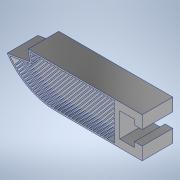
# Autodesk Inventor part: Finray_9_Kerbe_10deg
Saved by Autodesk Inventor 2022 (Build 260153000, 153)
## iProperties
Created: 2022-02-28
Part Number: Finray_9_Kerbe_10deg
Material: Generic
Document SubType Name: Modeling
Designer: richa
Density: 1 g/cm^3
Appearance: Aluminum - Flat
Author: richa
Autodesk Inventor part; units mm, degrees
ref_plane "YZ Plane" through (0, 0, 0) normal (1, 0, 0) x (0, 1, 0)
ref_plane "XZ Plane" through (0, 0, 0) normal (0, 1, 0) x (-1, 0, 0)
ref_plane "XY Plane" through (0, 0, 0) normal (0, 0, 1) x (1, 0, 0)
sketch "Sketch5" plane through (0, 0, 0) normal (0, 0, 1) x (1, 0, 0)
  line L0 (52.8, -15.6) -> (52.8, -10.6)
  line L1 (52.8, -10.6) -> (49.8, -10.6)
  line L2 (49.8, -10.6) -> (49.8, -12.6)
  line L3 (44, -12.6) -> (44, -3)
  line L4 (49.8, -3) -> (49.8, -5)
  line L5 (49.8, -5) -> (52.8, -5)
  line L6 (52.8, -5) -> (52.8, 0)
  line L7 (52.8, 0) -> (7.8, 0)
  line L8 (44, -3) -> (49.8, -3)
  line L9 (44, -12.6) -> (49.8, -12.6)
  line L10 (52.8, -15.6) -> (7.8, -15.6)
  line L11 (7.8, -15.6) -> (0, -15.6)
  line L12 (0, -15.6) -> (0, 0)
  line L13 (0, 0) -> (7.8, 0)
  point P0 (7.8, 0)
  dimension "d41" = 5.8
  dimension "d48" = 44
  dimension "d50" = 3
  dimension "d63" = 45
  dimension "d71" = 0
  dimension "d87" = 5.6
  dimension "d88" = 9.6
  dimension "d97" = 15.6
  constraints: 28 end point, 8 perpendicular, 4 collinear, 3 parallel, 2 horizontal, 1 vertical
  measures "d41" distance between parallel lines of L2 L3
  measures "d48" distance from line of L3 L12.end
  measures "d50" distance of L4.end L5.end
  measures "d63" distance of L0.start L10.end
  measures "d71" distance from line of L12.end L7
  measures "d87" distance from line of L0.end L5
  measures "d88" distance of L3.start L3.end
  measures "d97" distance of L11.end L12.end
extrude "Extrusion2" add sketch "Sketch5" along normal blind 12
sketch "Sketch8" plane through (0, 0, 0) normal (0, 0, -1) x (-1, 0, 0)
  line L0 (-8.1687, 0) -> (-8.8633, -3.9392)
  line L1 (-7.8, 0) -> (-1.143, 0) construction
  line L2 (0, -5.5021) -> (-8.8633, -3.9392)
  line L3 (-7.8, 0) -> (-8.1687, 0)
  line L4 (0, 0) -> (0, -15.6) projected
  line L5 (-52.8, 0) -> (0, 0) projected
  line L6 (-7.8, 0) -> (0, 0)
  line L7 (0, 0) -> (0, -5.5021)
  dimension "d80" = 100
  dimension "d95" = 4
  dimension "d96" = 9
  constraints: 12 end point, 2 collinear, 2 perpendicular, 1 horizontal, 1 point on line
  measures "d80" angle of L0 L1
  measures "d95" distance of L0.start L0.end
  measures "d96" distance of L2.start L0.end
extrude "Extrusion5" cut sketch "Sketch8" against normal through all
fillet "Fillet2" radius 23 1 edges at (0, -15.6, 6)
shell "Shell1" thickness 0.62 removed faces 1 at (23.9679, -7.5131, 12)
sketch "Sketch13" plane through (0, 0, 12) normal (0, 0, 1) x (1, 0, 0)
  line L0 (19.0404, -15.6) -> (52.8, -15.6) projected
  line L1 (42.0526, -15.6) -> (42.0526, 0)
  line L2 (52.8, 0) -> (8.1687, 0) projected
  line L3 (52.8, 0) -> (8.1687, 0) projected
  line L4 (52.8, -5) -> (52.8, 0) projected
  line L5 (49.8, -5) -> (52.8, -5) projected
  line L6 (49.8, -3) -> (49.8, -5) projected
  line L7 (44, -3) -> (49.8, -3) projected
  line L8 (44, -12.6) -> (44, -3) projected
  line L9 (49.8, -12.6) -> (44, -12.6) projected
  line L10 (49.8, -10.6) -> (49.8, -12.6) projected
  line L11 (52.8, -10.6) -> (49.8, -10.6) projected
  line L12 (52.8, -15.6) -> (52.8, -10.6) projected
  line L13 (42.0526, 0) -> (52.8, 0)
  line L14 (52.8, -5) -> (52.8, 0) projected
  line L15 (52.8, -5) -> (52.8, 0)
  line L16 (52.8, 0) -> (52.8, -5)
  line L17 (44, -12.6) -> (44, -3) projected
  line L18 (44, -3) -> (44, -12.6)
  line L19 (49.8, -12.6) -> (44, -12.6) projected
  line L20 (44, -12.6) -> (49.8, -12.6)
  line L21 (43.38, -13.22) -> (50.42, -13.22) projected
  line L22 (52.8, -10.6) -> (52.8, -15.6)
  line L23 (52.8, -15.6) -> (42.0526, -15.6)
  line L24 (44, -3) -> (49.8, -3) projected
  line L25 (44, -3) -> (49.8, -3)
  line L26 (49.8, -3) -> (49.8, -5)
  line L27 (49.8, -5) -> (52.8, -5)
  line L28 (52.8, -10.6) -> (49.8, -10.6)
  line L29 (49.8, -10.6) -> (49.8, -12.6)
  point P0 (0, 0)
  dimension "d102" = 10.7474
  constraints: 26 end point, 10 collinear, 2 point on line, 2 vertical, 1 parallel
  measures "d102" distance between parallel lines of L4 L1
extrude "Extrusion7" add sketch "Sketch13" against normal blind 12
sketch "Sketch14" plane through (8.9076, -0.62, 0.62) normal (0, 0, 1) x (1, 0, 0)
  line L0 (33.145, -14.36) -> (33.145, 0) projected
  line L1 (33.145, 0) -> (0, 0) projected
  line L2 (0.6739, -3.8221) -> (0, 0) projected
  line L3 (-7.835, -5.3225) -> (0.6739, -3.8221) projected
  arc A0 (-7.835, -5.3225) -> (10.1328, -14.36) centre (10.1328, 8.02) ccw projected
  line L4 (10.1328, -14.36) -> (33.145, -14.36) projected
  point P0 (-8.9076, 0.62)
extrude "Extrusion8" cut sketch "Sketch14" against normal blind 12
sketch "Sketch15" plane through (0, 0, 12) normal (0, 0, 1) x (1, 0, 0)
  line L0 (42.0526, -0.62) -> (8.9076, -0.62) construction
  line L1 (19.0404, -14.98) -> (42.0526, -14.98) projected
  line L2 (48.3066, -0.62) -> (36.2572, -14.98)
  line L3 (35.7611, -14.98) -> (47.8106, -0.62)
  line L4 (44.1485, -0.62) -> (32.099, -14.98)
  line L5 (31.6029, -14.98) -> (43.6524, -0.62)
  line L6 (39.9903, -0.62) -> (27.9408, -14.98)
  line L7 (27.4448, -14.98) -> (39.4943, -0.62)
  line L8 (35.8321, -0.62) -> (23.7827, -14.98)
  line L9 (23.2866, -14.98) -> (35.3361, -0.62)
  line L10 (31.674, -0.62) -> (19.6245, -14.98)
  line L11 (19.1285, -14.98) -> (31.1779, -0.62)
  line L12 (27.5158, -0.62) -> (15.6793, -14.7262)
  line L13 (15.2426, -14.6554) -> (27.0198, -0.62)
  line L14 (23.3577, -0.62) -> (11.7759, -14.4226)
  line L15 (19.1995, -0.62) -> (8.6931, -13.141)
  line L16 (8.3466, -12.9628) -> (18.7034, -0.62)
  arc A0 (1.0726, -5.9425) -> (19.0404, -14.98) centre (19.0404, 7.4) ccw projected
  line L17 (42.0526, -0.62) -> (42.0526, -14.98) projected
  line L18 (1.0726, -5.9425) -> (9.5815, -4.4421) projected
  arc A1 (0, -5.5021) -> (19.0404, -15.6) centre (19.0404, 7.4) ccw projected
  line L19 (10.3871, -0.62) -> (3.5571, -8.7596)
  line L20 (3.8342, -9.0206) -> (10.8832, -0.62)
  line L21 (14.5453, -0.62) -> (6.0082, -10.7941)
  line L22 (6.3201, -11.0135) -> (15.0413, -0.62)
  line L23 (42.0526, -14.98) -> (19.0404, -14.98) projected
  line L24 (38.5332, -14.98) -> (38.8243, -15.2243)
  line L25 (38.8243, -15.2243) -> (51.0787, -0.62)
  line L26 (51.0787, -0.62) -> (50.5827, -0.62)
  line L27 (50.5827, -0.62) -> (38.5332, -14.98)
  line L28 (8.9076, -0.62) -> (42.0526, -0.62) projected
  line L29 (46.4245, -0.62) -> (46.9206, -0.62)
  line L30 (46.9206, -0.62) -> (34.8711, -14.98)
  line L31 (34.8711, -14.98) -> (34.3751, -14.98)
  line L32 (34.3751, -14.98) -> (46.4245, -0.62)
  line L33 (42.2664, -0.62) -> (42.7624, -0.62)
  line L34 (42.7624, -0.62) -> (30.7129, -14.98)
  line L35 (30.7129, -14.98) -> (30.2169, -14.98)
  line L36 (30.2169, -14.98) -> (42.2664, -0.62)
  line L37 (38.1082, -0.62) -> (38.6043, -0.62)
  line L38 (38.6043, -0.62) -> (26.5548, -14.98)
  line L39 (26.5548, -14.98) -> (26.0587, -14.98)
  line L40 (26.0587, -14.98) -> (38.1082, -0.62)
  line L41 (33.95, -0.62) -> (34.4461, -0.62)
  line L42 (34.4461, -0.62) -> (22.3966, -14.98)
  line L43 (22.3966, -14.98) -> (21.9006, -14.98)
  line L44 (21.9006, -14.98) -> (33.95, -0.62)
  line L45 (29.7919, -0.62) -> (30.2879, -0.62)
  line L46 (30.2879, -0.62) -> (18.2385, -14.98)
  line L47 (18.2385, -14.98) -> (17.7424, -14.98)
  line L48 (17.7424, -14.98) -> (29.7919, -0.62)
  line L49 (25.6337, -0.62) -> (26.1298, -0.62)
  line L50 (26.1298, -0.62) -> (14.4751, -14.5094)
  line L51 (14.4751, -14.5094) -> (13.9791, -14.5094)
  line L52 (13.9791, -14.5094) -> (25.6337, -0.62)
  line L53 (21.4755, -0.62) -> (21.9716, -0.62)
  line L54 (21.9716, -0.62) -> (11.1333, -13.5366)
  line L55 (11.1333, -13.5366) -> (10.6372, -13.5366)
  line L56 (10.6372, -13.5366) -> (21.4755, -0.62)
  line L57 (17.3174, -0.62) -> (17.8134, -0.62)
  line L58 (17.8134, -0.62) -> (8.1413, -12.1467)
  line L59 (8.1413, -12.1467) -> (7.6453, -12.1467)
  line L60 (7.6453, -12.1467) -> (17.3174, -0.62)
  line L61 (9.4971, -0.62) -> (3.0705, -8.2789)
  line L62 (2.8052, -8.004) -> (9.001, -0.62)
  line L63 (10.5986, -4.2628) -> (10.1025, -4.2628)
  line L64 (13.1592, -0.62) -> (5.1587, -10.1546)
  line L65 (5.459, -10.3879) -> (13.6553, -0.62)
  line L66 (49.1966, -0.62) -> (49.6927, -0.62)
  line L67 (49.6927, -0.62) -> (37.6432, -14.98)
  line L68 (37.6432, -14.98) -> (37.1472, -14.98)
  line L69 (37.1472, -14.98) -> (49.1966, -0.62)
  line L70 (45.0385, -0.62) -> (45.5345, -0.62)
  line L71 (45.5345, -0.62) -> (33.4851, -14.98)
  line L72 (33.4851, -14.98) -> (32.989, -14.98)
  line L73 (32.989, -14.98) -> (45.0385, -0.62)
  line L74 (40.8803, -0.62) -> (41.3764, -0.62)
  line L75 (41.3764, -0.62) -> (29.3269, -14.98)
  line L76 (29.3269, -14.98) -> (28.8308, -14.98)
  line L77 (28.8308, -14.98) -> (40.8803, -0.62)
  line L78 (36.7221, -0.62) -> (37.2182, -0.62)
  line L79 (37.2182, -0.62) -> (25.1687, -14.98)
  line L80 (25.1687, -14.98) -> (24.6727, -14.98)
  line L81 (24.6727, -14.98) -> (36.7221, -0.62)
  line L82 (32.564, -0.62) -> (33.06, -0.62)
  line L83 (33.06, -0.62) -> (21.0106, -14.98)
  line L84 (21.0106, -14.98) -> (20.5145, -14.98)
  line L85 (20.5145, -14.98) -> (32.564, -0.62)
  line L86 (28.4058, -0.62) -> (28.9019, -0.62)
  line L87 (28.9019, -0.62) -> (16.8524, -14.98)
  line L88 (16.8524, -14.98) -> (16.3563, -14.98)
  line L89 (16.3563, -14.98) -> (28.4058, -0.62)
  line L90 (24.2477, -0.62) -> (24.7437, -0.62)
  line L91 (24.7437, -0.62) -> (13.3184, -14.2362)
  line L92 (13.3184, -14.2362) -> (12.8223, -14.2362)
  line L93 (12.8223, -14.2362) -> (24.2477, -0.62)
  line L94 (20.0895, -0.62) -> (20.5855, -0.62)
  line L95 (20.5855, -0.62) -> (10.0997, -13.1165)
  line L96 (10.0997, -13.1165) -> (9.6036, -13.1165)
  line L97 (9.6036, -13.1165) -> (20.0895, -0.62)
  line L98 (8.9718, -4.5497) -> (8.4758, -4.5497)
  line L99 (11.7732, -0.62) -> (4.3417, -9.4764)
  line L100 (4.6304, -9.7236) -> (12.2692, -0.62)
  line L101 (16.4274, -0.62) -> (15.9313, -0.62)
  line L102 (15.9313, -0.62) -> (6.8903, -11.3947)
  line L103 (7.214, -11.6) -> (16.4274, -0.62)
  line L104 (8.9076, -0.62) -> (-0.0004, -0.62) construction
  line L105 (47.8106, -0.62) -> (48.3066, -0.62)
  line L106 (11.8171, -13.7823) -> (22.8616, -0.62)
  point P0 (0, 0)
  point P1 (33.931, -17.161)
  point P2 (38.8393, -6.356)
  point P3 (29.043, -18.6221)
  point P4 (39.2193, -6.4943)
  point P5 (28.6321, -18.5205)
  point P6 (34.7397, -6.2863)
  point P7 (25.0778, -18.392)
  point P8 (24.4739, -18.5205)
  point P9 (27.5179, -9.9373)
  point P10 (28.1855, -9.733)
  point P11 (24.5233, -8.5506)
  point P12 (24.9033, -8.6889)
  point P13 (21.5288, -7.1639)
  point P14 (21.9088, -7.3022)
  point P15 (18.1464, -6.2394)
  point P16 (18.5264, -6.3777)
  point P17 (13.7227, -6.5558)
  point P18 (14.1901, -6.59)
  point P19 (7.3451, -4.8365)
  point P20 (4.128, -8.0793)
  point P21 (4.3811, -12.7332)
  point P22 (4.8055, -12.8186)
  point P23 (35.7611, -14.98)
  point P24 (31.6029, -14.98)
  point P25 (32.099, -14.98)
  point P26 (29.4219, -14.98)
  point P27 (27.9408, -14.98)
  point P28 (25.0643, -14.98)
  point P29 (23.7827, -14.98)
  point P30 (20.6649, -14.98)
  point P31 (21.1037, -14.98)
  point P32 (19.6462, -14.98)
  point P33 (20.0321, -14.98)
  point P34 (8.7548, -12.4764)
  point P35 (9.1029, -12.6527)
  point P36 (5.1362, -5.226)
  point P37 (3.0438, -8.3108)
  point P38 (1.8569, -9.134)
  point P39 (6.3464, -8.7392)
  point P40 (6.7558, -8.8424)
  point P41 (38.5332, -14.98)
  point P42 (39.0293, -14.98)
  point P43 (34.3751, -14.98)
  point P44 (34.8711, -14.98)
  point P45 (41.7215, -0.62)
  point P46 (41.1434, -0.62)
  point P47 (30.7129, -14.98)
  point P48 (41.6394, -0.62)
  point P49 (38.1082, -0.62)
  point P50 (26.5548, -14.98)
  point P51 (38.6043, -0.62)
  point P52 (33.95, -0.62)
  point P53 (22.3966, -14.98)
  point P54 (34.4461, -0.62)
  point P55 (29.7919, -0.62)
  point P56 (19.1984, -14.98)
  point P57 (19.0819, -14.98)
  point P58 (30.2879, -0.62)
  point P59 (26.1298, -0.62)
  point P60 (21.9716, -0.62)
  point P61 (17.8134, -0.62)
  point P62 (3.8395, -10.0749)
  point P63 (4.3026, -10.1142)
  point P64 (4.8631, -13.8106)
  point P65 (5.3932, -13.77)
  point P66 (37.6432, -14.98)
  point P67 (40.9208, -0.62)
  point P68 (32.989, -14.98)
  point P69 (33.4851, -14.98)
  point P70 (40.3355, -0.62)
  point P71 (29.3269, -14.98)
  point P72 (41.3764, -0.62)
  point P73 (25.1687, -14.98)
  point P74 (37.2182, -0.62)
  point P75 (21.0106, -14.98)
  point P76 (33.06, -0.62)
  point P77 (19.6871, -14.98)
  point P78 (19.1528, -14.98)
  point P79 (28.9019, -0.62)
  point P80 (24.7437, -0.62)
  point P81 (20.5855, -0.62)
  point P82 (15.9313, -0.62)
  point P83 (5.7184, -5.1233)
  point P84 (6.7629, -4.9391)
  point P85 (8.3897, -4.6523)
  point P86 (8.6984, -4.5979)
  point P87 (6.1234, -5.0519)
  point P88 (5.5412, -5.1546)
  point P89 (12.2054, -13.9107)
  point P90 (15.0413, -0.62)
  point P91 (14.5453, -0.62)
  point P92 (13.6553, -0.62)
  point P93 (13.1592, -0.62)
  point P94 (17.1982, -15.5261)
  point P95 (17.5923, -15.5544)
  point P96 (27.0198, -0.62)
  point P97 (16.3586, -14.8187)
  point P98 (16.7709, -14.8646)
  point P99 (42.0526, -3.1178)
  point P100 (42.0526, -2.5266)
  point P101 (10.8832, -0.62)
  point P102 (10.3871, -0.62)
  point P103 (12.2692, -0.62)
  point P104 (11.7732, -0.62)
  dimension "d105" = 0.38
  dimension "d107" = 0.38
  dimension "d110" = 0.38
  dimension "d111" = 0.38
  dimension "d113" = 0.38
  dimension "d129" = 0.38
  dimension "d131" = 0.38
  dimension "d132" = 0.38
  dimension "d133" = 0.38
  dimension "d134" = 0.38
  dimension "d135" = 0.38
  dimension "d136" = 0.38
  dimension "d137" = 0.38
  dimension "d138" = 0.38
  dimension "d139" = 0.38
  dimension "d151" = 0.38
  dimension "d157" = 0.38
  dimension "d161" = 0.38
  dimension "d163" = 0.38
  dimension "d169" = 0.38
  dimension "d172" = 0.38
  dimension "d175" = 0.38
  dimension "d185" = 130
  dimension "d186" = 130
  dimension "d187" = 130
  dimension "d189" = 0.89
  dimension "d200" = 0.38
  dimension "d201" = 130
  dimension "d202" = 0.89
  dimension "d205" = 0.89
  dimension "d206" = 0.89
  dimension "d207" = 0.89
  dimension "d209" = 0.89
  dimension "d210" = 0.38
  dimension "d211" = 0.38
  dimension "d213" = 0.89
  dimension "d214" = 0.38
  dimension "d215" = 0.38
  dimension "d216" = 0.38
  dimension "d217" = 0.89
  dimension "d218" = 0.89
  dimension "d221" = 0.89
  dimension "d222" = 0.89
  dimension "d223" = 0.89
  dimension "d224" = 0.38
  dimension "d225" = 0.89
  dimension "d226" = 0.89
  dimension "d227" = 0.89
  dimension "d228" = 0.89
  dimension "d229" = 0.89
  dimension "d232" = 0.38
  dimension "d233" = 0.89
  dimension "d234" = 0.89
  dimension "d235" = 0.38
  dimension "d236" = 0.89
  dimension "d237" = 0.89
  dimension "d238" = 0.89
  dimension "d239" = 0.89
  dimension "d240" = 0.89
  dimension "d241" = 0.89
  dimension "d242" = 0.89
  dimension "d243" = 0.89
  dimension "d244" = 0.89
  dimension "d245" = 0.89
  constraints: 200 end point, 70 parallel, 45 point on line, 20 horizontal, 3 point on circle, 1 collinear, 1 perpendicular, 85 other
  measures "d105" distance between parallel lines of L2 L3
  measures "d107" distance between parallel lines of L4 L5
  measures "d110" distance between parallel lines of L10 L11
  measures "d111" distance between parallel lines of L12 L13
  measures "d113" distance between parallel lines of L15 L16
  measures "d129" distance between parallel lines of L25 L27
  measures "d131" distance between parallel lines of L30 L32
  measures "d132" distance between parallel lines of L34 L36
  measures "d133" distance between parallel lines of L38 L40
  measures "d134" distance between parallel lines of L42 L44
  measures "d135" distance between parallel lines of L46 L48
  measures "d136" distance between parallel lines of L50 L52
  measures "d137" distance between parallel lines of L54 L56
  measures "d138" distance between parallel lines of L58 L60
  measures "d139" distance between parallel lines of L65 L64
  measures "d151" distance between parallel lines of L67 L69
  measures "d157" distance between parallel lines of L71 L73
  measures "d161" distance between parallel lines of L75 L77
  measures "d163" distance between parallel lines of L79 L81
  measures "d169" distance between parallel lines of L87 L89
  measures "d172" distance between parallel lines of L91 L93
  measures "d175" distance between parallel lines of L95 L97
  measures "d185" angle to the sketch x axis of L25
  measures "d186" angle of L0 L30
  measures "d187" angle of L0 L2
  measures "d189" distance of L33.start L74.end
  measures "d200" distance between parallel lines of L83 L85
  measures "d201" angle of L0 L91
  measures "d202" distance of L101.end L22.end
  measures "d205" distance of L29.start L70.end
  measures "d206" distance of L3.end L29.end
  measures "d207" distance of L66.start L2.start
  measures "d209" distance of L26.end L66.end
  measures "d210" distance between parallel lines of L22 L21
  measures "d211" distance between parallel lines of L14 L106
  measures "d213" distance of L21.start L65.end
  measures "d214" distance between parallel lines of L100 L99
  measures "d215" distance between parallel lines of L19 L20
  measures "d216" distance between parallel lines of L62 L61
  measures "d217" distance of L99.start L20.end
  measures "d218" distance of L19.start L61.start
  measures "d221" distance of L94.start L15.start
  measures "d222" distance of L106.end L53.end
  measures "d223" distance of L90.start L14.start
  measures "d224" distance between parallel lines of L6 L7
  measures "d225" distance of L4.start L70.start
  measures "d226" distance of L33.end L5.end
  measures "d227" distance of L7.end L37.end
  measures "d228" distance of L74.start L6.start
  measures "d229" distance of L37.start L78.end
  measures "d232" distance between parallel lines of L8 L9
  measures "d233" distance of L57.start L101.start
  measures "d234" distance of L64.start L100.end
  measures "d235" distance between parallel lines of L103 L102
  measures "d236" distance of L16.end L57.end
  measures "d237" distance of L53.start L94.end
  measures "d238" distance of L49.start L90.end
  measures "d239" distance of L13.end L49.end
  measures "d240" distance of L86.start L12.start
  measures "d241" distance of L86.end L45.start
  measures "d242" distance of L45.end L11.end
  measures "d243" distance of L82.start L10.start
  measures "d244" distance of L82.end L41.start
  measures "d245" distance of L41.end L9.end
extrude "Extrusion9" add sketch "Sketch15" against normal blind 12 contours L11 L28 L10 L1 | L46 L47 L48 A0 | A0 L48 L28 L46 | L85 L28 L83 L1 | L87 L88 L89 A0 | A0 L89 L28 L87 | L44 L28 L42 L1 | A0 L13 L28 L12 | L9 L28 L8 L1 | L51 L52 A0 | A0 L52 L28 L50 | L81 L28 L79 L1 | L92 L93 A0 | A0 L93 L28 L91 | L40 L28 L38 L1 | A0 L106 L28 L14 | L7 L28 L6 L1 | L55 L56 A0 | A0 L56 L28 L54 | A0 L16 L28 L15 | L77 L28 L75 L1 | L97 L28 L95 A0 | A0 L96 L97 | L59 L60 A0 | A0 L60 L28 L58 | L36 L17 L34 L1 | L36 L33 L34 L17 | A0 L102 L28 L103 | L5 L17 L4 L1 | A0 L21 L28 L22 | L73 L17 L71 L1 | L73 L70 L71 L17 | A0 L64 L63 L65 | L32 L17 L30 L1 | L65 L63 L64 L28 | L32 L29 L30 L17 | A0 L99 L18 L100 | L3 L17 L2 L1 | L100 L98 L99 L28 | L18 L99 L98 | L3 L105 L2 L17 | A0 L19 L18 L20 | L69 L17 L67 L1 | L20 L18 L19 L28 | L69 L66 L67 L17 | A0 L62 L18 L61 | L27 L17 L25 L1 | L27 L26 L25 L17
sketch "Sketch16" plane through (0, 0, 12) normal (0, 0, 1) x (1, 0, 0)
  arc A0 (0, -5.5021) -> (19.0404, -15.6) centre (19.0404, 7.4) ccw projected
  line L0 (9.5815, -4.4421) -> (8.9076, -0.62) projected
  line L1 (8.1687, 0) -> (8.8633, -3.9392) projected
  line L2 (8.1687, 0) -> (8.8633, -3.9392)
  line L3 (52.8, 0) -> (8.1687, 0) projected
  line L4 (0, -5.5021) -> (8.1687, 0)
  line L5 (0, -5.5021) -> (8.8633, -3.9392)
  point P0 (0, 0)
  point P1 (9.3319, -3.0264)
  point P2 (8.8242, -3.7175)
  point P3 (8.8303, -3.7523)
  point P4 (9.4967, -3.9613)
  point P5 (9.441, -3.645)
  point P6 (8.8303, -3.7523)
  constraints: 6 end point, 1 collinear, 1 perpendicular
extrude "Extrusion10" cut sketch "Sketch16" against normal blind 12
sketch "Sketch17" plane through (0, 0, 12) normal (0, 0, 1) x (1, 0, 0)
  line L0 (49.8, -12.6) -> (44, -12.6) projected
  line L1 (49.8, -3) -> (49.8, -5) projected
  line L2 (44, -12.6) -> (49.8, -12.6)
  line L3 (49.8, -12.6) -> (49.8, -3)
  line L4 (49.8, -3) -> (44, -3)
  line L5 (44, -3) -> (44, -12.6)
  point P0 (0, 0)
  constraints: 8 end point, 2 parallel, 1 horizontal, 1 perpendicular
extrude "Extrusion11" cut sketch "Sketch17" against normal blind 12
equation "\"l1\" = 8"
equation "\"d1\" = 0.38"
body "Solid2"
